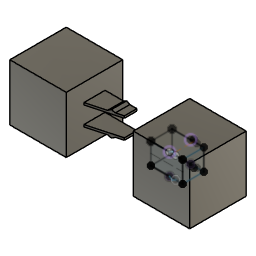
LockIn Tabs tryout v4 (Autodesk Fusion 360 design; units mm, degrees)
Autodesk Fusion 360 part; units mm, degrees
sketch "Sketch1" plane through (0, 0, 0) normal (0, 1, 0) x (1, 0, 0)
  line L0 (-100, 0) -> (-20, 0)
  line L1 (-20, 0) -> (-20, -80)
  line L2 (-20, -80) -> (-100, -80)
  line L3 (-100, -80) -> (-100, 0)
  line L4 (75, 0) -> (155, 0)
  line L5 (155, 0) -> (155, -80)
  line L6 (155, -80) -> (75, -80)
  line L7 (75, -80) -> (75, 0)
  dimension "d1" = 80
  dimension "d2" = 80
  dimension "d3" = 80
  dimension "d4" = 80
  constraint horizontal L0
  constraint vertical L1
  constraint horizontal L2
  constraint vertical L3
  constraint horizontal L4
  constraint vertical L5
  constraint horizontal L6
  constraint vertical L7
  measures "d1" distance of L0.start L0.end
  measures "d2" distance of L0.start L2.end
  measures "d3" distance of L4.start L4.end
  measures "d4" distance of L4.start L6.end
extrude "Extrude1" add sketch "Sketch1" along normal blind 80 contours L0 L1 L2 L3 makes body 1
extrude "Extrude2" add sketch "Sketch1" along normal blind 80 separate body contours L4 L5 L6 L7 makes body 2
sketch "Sketch2" plane through (75, 0, 0) normal (-1, 0, 0) x (0, -1, 0)
  line L0 (0, 0) -> (0, 80)
  line L1 (0, 80) -> (-80, 80)
  line L2 (-80, 80) -> (-80, 0)
  line L3 (-80, 0) -> (0, 0)
  line L4 (-55, 25) -> (-25, 25)
  line L5 (-25, 25) -> (-25, 55)
  line L6 (-25, 55) -> (-55, 55)
  line L7 (-55, 55) -> (-55, 25)
  constraint horizontal L4
  constraint vertical L5
  constraint horizontal L6
  constraint vertical L7
extrude "Extrude3" cut sketch "Sketch2" against normal blind 45 contours L4 L5 L6 L7 bodies 2
sketch "Sketch3" plane through (0, 0, 0) normal (0, -1, 0) x (1, 0, 0)
  line L0 (155, 80) -> (75, 80)
  line L1 (75, 80) -> (75, 0)
  line L2 (75, 0) -> (155, 0)
  line L3 (155, 0) -> (155, 80)
  line L4 (75, 40) -> (155, 40) construction
  line L5 (75, 40) -> (75, 25) construction
  line L6 (75, 40) -> (75, 55) construction
  line L7 (75, 55) -> (120, 55) construction
  line L8 (120, 55) -> (120, 25) construction
  line L9 (120, 25) -> (75, 25) construction
  line L10 (75, 55) -> (120, 55)
  line L11 (120, 25) -> (75, 25)
  line L12 (120, 55) -> (110, 55) construction
  line L13 (110, 55) -> (110, 60) construction
  line L14 (110, 55) -> (105.6699, 57.5)
  line L15 (110, 55) -> (115, 55) construction
  line L16 (105.6699, 57.5) -> (101.3397, 55)
  line L17 (105.6699, 22.5) -> (101.3397, 25)
  line L18 (110, 25) -> (105.6699, 22.5)
  dimension "d11" = 150
  dimension "d12" = 5
  constraint midpoint L1 L4.start
  constraint midpoint L3 L4.end
  constraint coincident L1 L5.end
  constraint perpendicular L4 L5
  constraint coincident L1 L6.end
  constraint perpendicular L4 L6
  constraint perpendicular L6 L7
  constraint perpendicular L4 L8
  constraint perpendicular L5 L9
  constraint coincident L7 L12.end
  constraint perpendicular L12 L13
  constraint horizontal L15
  constraint coincident L10 L16.end
  constraint symmetric L4 L12.end L18.start
  constraint symmetric L4 L14.end L17.start
  constraint symmetric L4 L16.end L17.end
  measures "d11" angle of L14 L15
  measures "d12" distance of L14.end L16.end
sketch "Sketch4" plane through (0, 25, 0) normal (0, 1, 0) x (-1, 0, 0)
  line L0 (-75, 25) -> (-75, 55)
  line L1 (-75, 55) -> (-120, 55)
  line L2 (-120, 55) -> (-120, 25)
  line L3 (-120, 25) -> (-75, 25)
  line L4 (-75, 40) -> (-120, 40) construction
  line L5 (-120, 40) -> (-120, 55) construction
  line L6 (-120, 55) -> (-75, 55) construction
  line L7 (-120, 40) -> (-120, 25) construction
  line L8 (-120, 25) -> (-75, 25)
  line L9 (-110, 25) -> (-105.6699, 22.5)
  line L10 (-105.6699, 22.5) -> (-101.3397, 25)
  line L11 (-105.6699, 57.5) -> (-101.3397, 55)
  line L12 (-110, 55) -> (-105.6699, 57.5)
  dimension "d13" = 150
  dimension "d14" = 5
  dimension "d15" = 5
  constraint midpoint L0 L4.start
  constraint midpoint L2 L4.end
  constraint coincident L1.end L2.start
  constraint coincident L0.end L1.start
  constraint coincident L2.end L3.start
  constraint coincident L0.start L3.end
  constraint coincident L3 L9.start
  constraint coincident L8 L10.end
  constraint symmetric L4 L9.start L12.start
  constraint symmetric L4 L9.end L11.start
  constraint symmetric L4 L10.end L11.end
  measures "d13" angle of L8 L9
  measures "d14" distance of L9.start L9.end
  measures "d15" distance of L9.end L10.end
extrude "Extrude4" cut sketch "Sketch4" along normal up to surface (30 mm away) contours L3 L8 L9 L10 | L1 L11 L12 bodies 2
sketch "Sketch5" plane through (0, 0, 25) normal (0, 0, 1) x (-1, 0, 0)
  line L0 (-101.3397, -55) -> (-75, -55)
  line L1 (-75, -55) -> (-75, -25)
  line L2 (-75, -25) -> (-101.3397, -25)
  line L3 (-101.3397, -55) -> (-75, -55)
  line L4 (-75, -55) -> (-75, -25)
  line L5 (-75, -25) -> (-101.3397, -25)
  line L6 (-110, -55) -> (-120, -55)
  line L7 (-120, -55) -> (-120, -25)
  line L8 (-120, -25) -> (-110, -25)
  line L9 (-101.3397, -55) -> (-110, -55)
  line L10 (-110, -25) -> (-101.3397, -25)
  constraint coincident L0.start L3.start
  constraint coincident L0.end L1.start
  constraint coincident L1.end L2.start
  constraint coincident L2.end L5.end
  constraint perpendicular L6 L7
sketch "Sketch6" plane through (120, 0, 0) normal (-1, 0, 0) x (0, -1, 0)
  line L0 (-55, 55) -> (-55, 25)
  line L1 (-55, 25) -> (-25, 25)
  line L2 (-25, 25) -> (-25, 55)
  line L3 (-25, 55) -> (-55, 55)
  line L4 (-25, 25) -> (-25, 55)
  line L5 (-25, 55) -> (-55, 55)
  line L6 (-55, 55) -> (-55, 25)
  line L7 (-55, 25) -> (-25, 25)
  constraint coincident L1.end L2.start
  constraint coincident L2.end L3.start
  constraint coincident L0.start L3.end
  constraint coincident L0.end L1.start
sketch "Sketch7" plane through (0, 25, 0) normal (0, 1, 0) x (-1, 0, 0)
  line L0 (-75, 25) -> (-75, 55)
  line L1 (-75, 55) -> (-101.3397, 55)
  line L2 (-101.3397, 55) -> (-105.6699, 57.5)
  line L3 (-105.6699, 57.5) -> (-110, 55)
  line L4 (-110, 55) -> (-120, 55)
  line L5 (-120, 55) -> (-120, 25)
  line L6 (-120, 25) -> (-110, 25)
  line L7 (-110, 25) -> (-105.6699, 22.5)
  line L8 (-105.6699, 22.5) -> (-101.3397, 25)
  line L9 (-101.3397, 25) -> (-75, 25)
  line L10 (-120, 55) -> (-75, 55)
  line L11 (-75, 55) -> (-75, 25)
  line L12 (-120, 25) -> (-75, 25)
  line L13 (-120, 25) -> (-120, 55)
  constraint coincident L4.end L5.start
  constraint coincident L0.end L1.start
  constraint coincident L0.start L9.end
  constraint coincident L5.end L6.start
sketch "Sketch8" plane through (0, 55, 0) normal (0, -1, 0) x (1, 0, 0)
  line L0 (75, 55) -> (75, 25)
  line L1 (75, 25) -> (101.3397, 25)
  line L2 (101.3397, 25) -> (105.6699, 22.5)
  line L3 (105.6699, 22.5) -> (110, 25)
  line L4 (110, 25) -> (120, 25)
  line L5 (120, 25) -> (120, 55)
  line L6 (120, 55) -> (110, 55)
  line L7 (110, 55) -> (105.6699, 57.5)
  line L8 (105.6699, 57.5) -> (101.3397, 55)
  line L9 (101.3397, 55) -> (75, 55)
  line L10 (120, 55) -> (120, 25)
  line L11 (120, 25) -> (75, 25)
  line L12 (120, 55) -> (75, 55)
  line L13 (75, 55) -> (75, 25)
  line L14 (101.3397, 25) -> (105.6699, 22.5)
  line L15 (110, 25) -> (105.6699, 22.5)
  line L16 (110, 55) -> (105.6699, 57.5)
  line L17 (105.6699, 57.5) -> (101.3397, 55)
  constraint coincident L5.end L6.start
  constraint coincident L4.end L5.start
  constraint coincident L0.end L1.start
  constraint coincident L0.start L9.end
  constraint coincident L1.end L2.start
  constraint coincident L2.end L3.start
  constraint coincident L3.end L4.start
  constraint coincident L6.end L7.start
  constraint coincident L7.end L8.start
  constraint coincident L8.end L9.start
sketch "Sketch9" plane through (0, 0, 55) normal (0, 0, -1) x (1, 0, 0)
  line L0 (101.3397, -25) -> (75, -25)
  line L1 (75, -25) -> (75, -55)
  line L2 (75, -55) -> (101.3397, -55)
  line L3 (75, -55) -> (120, -55)
  line L4 (75, -55) -> (75, -25)
  line L5 (120, -55) -> (120, -25)
  line L6 (120, -25) -> (75, -25)
  line L7 (110, -55) -> (105.67, -55)
  line L8 (105.67, -55) -> (105.67, -25) construction
  dimension "d19" = 4.33
  constraint coincident L1.end L2.start
  constraint perpendicular L1 L3
  constraint coincident L0.end L1.start
  constraint perpendicular L3 L5
  constraint perpendicular L4 L6
  constraint coincident L3 L7.start
  constraint parallel L2 L7
  constraint coincident L6 L8.end
  constraint perpendicular L6 L8
  measures "d19" distance of L7.start L7.end
sketch "Sketch10" plane through (-20, 0, 0) normal (1, 0, 0) x (0, 1, 0)
  line L0 (0, 80) -> (0, 0)
  line L1 (0, 0) -> (80, 0)
  line L2 (80, 0) -> (80, 80)
  line L3 (80, 80) -> (0, 80)
  line L4 (55, 55) -> (25, 55)
  line L5 (25, 25) -> (55, 25)
  line L6 (25, 55) -> (25, 52)
  line L7 (25, 52) -> (55, 52)
  line L8 (55, 52) -> (55, 55)
  line L9 (25, 25) -> (25, 28)
  line L10 (25, 28) -> (55, 28)
  line L11 (55, 28) -> (55, 25)
  dimension "d20" = 3
  dimension "d21" = 3
  constraint horizontal L4
  constraint horizontal L5
  constraint perpendicular L4 L6
  constraint perpendicular L6 L7
  constraint perpendicular L4 L8
  constraint perpendicular L5 L9
  constraint perpendicular L9 L10
  constraint perpendicular L5 L11
  measures "d20" distance of L4.end L6.end
  measures "d21" distance of L5.start L9.end
extrude "Extrude5" add sketch "Sketch10" along normal blind 45 contours L4 L6 L7 L8 | L5 L9 L10 L11 bodies 1
sketch "Sketch11" plane through (0, 25, 0) normal (0, -1, 0) x (1, 0, 0)
  line L0 (-20, 55) -> (-20, 52)
  line L1 (-20, 52) -> (25, 52)
  line L2 (25, 52) -> (25, 55)
  line L3 (25, 55) -> (-20, 55)
  line L4 (25, 55) -> (15, 55)
  line L5 (15, 55) -> (10.6699, 57.5)
  line L6 (15, 55) -> (20, 55) construction
  line L7 (10.6699, 57.5) -> (6.3397, 55)
  line L8 (-20, 40) -> (25, 40) construction
  line L9 (15, 25) -> (10.6699, 22.5)
  line L10 (10.6699, 22.5) -> (6.3397, 25)
  dimension "d24" = 150
  dimension "d25" = 5
  dimension "d26" = 5
  constraint coincident L2.end L3.start
  constraint coincident L3 L4.end
  constraint perpendicular L2 L4
  constraint horizontal L6
  constraint coincident L3 L7.end
  constraint parallel L1 L8
  constraint symmetric L4.end L8 L9.start
  constraint symmetric L5.end L8 L9.end
  constraint symmetric L7.end L8 L10.end
  measures "d24" angle of L5 L6
  measures "d25" distance of L4.end L5.end
  measures "d26" distance of L5.end L7.end
extrude "Extrude6" add sketch "Sketch11" against normal blind 30 contours L3 L5 L7 bodies 1
sketch "Sketch12" plane through (0, 25, 0) normal (0, -1, 0) x (1, 0, 0)
  line L0 (-20, 28) -> (-20, 25)
  line L1 (-20, 25) -> (25, 25)
  line L2 (25, 25) -> (25, 28)
  line L3 (25, 28) -> (-20, 28)
  line L4 (25, 25) -> (15, 25)
  line L5 (15, 25) -> (10.6699, 22.5)
  line L6 (10.6699, 22.5) -> (6.3397, 25)
  dimension "d29" = 150
  dimension "d30" = 5
  dimension "d31" = 5
  constraint coincident L1.end L2.start
  constraint coincident L1 L4.end
  constraint perpendicular L2 L4
  constraint coincident L1 L6.end
  measures "d29" angle of L4 L5
  measures "d30" distance of L4.end L5.end
  measures "d31" distance of L5.end L6.end
extrude "Extrude7" add sketch "Sketch12" against normal blind 30 contours L1 L5 L6 bodies 1
sketch "Sketch13" plane through (0, 0, 0) normal (0, 0, 1) x (1, 0, 0)
  line L0 (-20, 25) -> (35, 40)
  line L1 (35, 40) -> (35, 20)
  line L2 (35, 20) -> (-20, 25)
  constraint vertical L1
extrude "Extrude8" cut sketch "Sketch13" along normal blind 70 bodies 1
equation "d19 = ( 8.660 / 2 ) * 1 mm"
